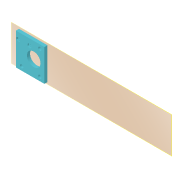
# Autodesk Inventor part: BallMountRight
Saved by Autodesk Inventor 2018 (Build 220112000, 112)
## iProperties
Created: 2019-02-16
Part Number: BallMountRight
Material: Generic
Document SubType Name: Modeling
Designer: ball
Density: 1 g/cm^3
Appearance: Default
Author: ball
Autodesk Inventor part; units mm, degrees
ref_plane "YZ Plane" through (0, 0, 0) normal (1, 0, 0) x (0, 1, 0)
ref_plane "XZ Plane" through (0, 0, 0) normal (0, 1, 0) x (-1, 0, 0)
ref_plane "XY Plane" through (0, 0, 0) normal (0, 0, 1) x (1, 0, 0)
ref_plane "Work Plane1" through (0, 0, 0) normal (0, 0, 1) x (1, 0, 0)
sketch "Sketch1" plane through (0, 0, 0) normal (0, 0, 1) x (1, 0, 0)
  line L0 (-192, 0) -> (-192, -43) construction
  line L1 (-192, -43) -> (0, -43) construction
  line L2 (-192, 0) -> (0, 0) construction
  line L3 (-153.9875, -0.508) -> (-153.9875, -42.492)
  line L4 (-153.9875, -42.492) -> (-191.492, -42.492)
  line L5 (-191.492, -42.492) -> (-191.492, -0.508)
  line L6 (-191.492, -0.508) -> (-153.9875, -0.508)
  circle A0 centre (-168, -21.5) radius 7.975 construction
  circle A1 centre (-168, -21.5) radius 8.89
  circle A2 centre (-184, -37.5) radius 2 construction
  circle A3 centre (-160, -37.5) radius 2 construction
  circle A4 centre (-160, -5.5) radius 2 construction
  circle A5 centre (-184, -37.5) radius 2.1844
  circle A6 centre (-160, -37.5) radius 2.1844
  circle A7 centre (-160, -5.5) radius 2.1844
extrude "Extrusion1" add sketch "Sketch1" along normal blind 4.064
sketch "Sketch2" plane through (0, 0, 4.064) normal (0, 0, 1) x (1, 0, 0)
  arc A0 (-188.6973, -7.9203) -> (-188.6973, -10.181) centre (-188.5276, -9.0507) ccw construction
  arc A1 (-173.6259, -10.181) -> (-173.6259, -7.9203) centre (-173.7956, -9.0507) ccw construction
  circle A2 centre (-188.5276, -9.0507) radius 1.3716
  circle A3 centre (-173.7956, -9.0507) radius 1.3716
  point P0 (0, 0)
  dimension "d7" = 2.7432
  dimension "d8" = 2.7432
  constraints: 2 centre point, 2 coincident
  measures "d7" diameter of A2
  measures "d8" diameter of A3
extrude "Extrusion2" cut sketch "Sketch2" against normal through all
sketch "Sketch4" plane through (0, 0, 4.064) normal (0, 0, 1) x (1, 0, 0)
  circle A0 centre (-188.5276, -9.0507) radius 1.3716 construction
  circle A1 centre (-188.5276, -9.0507) radius 2.794 construction
  circle A2 centre (-173.7956, -9.0507) radius 1.3716 construction
  circle A3 centre (-173.7956, -9.0507) radius 2.794 construction
  line L0 (-188.5276, -11.8447) -> (-190.9473, -10.4477)
  line L1 (-190.9473, -10.4477) -> (-190.9473, -7.6537)
  line L2 (-190.9473, -7.6537) -> (-188.5276, -6.2567)
  line L3 (-188.5276, -6.2567) -> (-186.108, -7.6537)
  line L4 (-186.108, -7.6537) -> (-186.108, -10.4477)
  line L5 (-186.108, -10.4477) -> (-188.5276, -11.8447)
  line L6 (-173.7956, -11.8447) -> (-176.2153, -10.4477)
  line L7 (-176.2153, -10.4477) -> (-176.2153, -7.6537)
  line L8 (-176.2153, -7.6537) -> (-173.7956, -6.2567)
  line L9 (-173.7956, -6.2567) -> (-171.376, -7.6537)
  line L10 (-171.376, -7.6537) -> (-171.376, -10.4477)
  line L11 (-171.376, -10.4477) -> (-173.7956, -11.8447)
  point P0 (0, 0)
  dimension "d15" = 5.588
  dimension "d16" = 5.588
  constraints: 24 end point, 4 coincident, 2 vertical alignment, 30 other
extrude "Extrusion4" cut sketch "Sketch4" against normal blind 2.032
body "Solid1"
